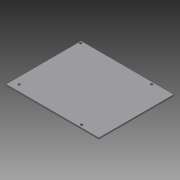
# Autodesk Inventor part: Smoothieboard
Saved by Autodesk Inventor 2014 (Build 180170000, 170)
## iProperties
Created: 2015-02-09
Part Number: Smoothieboard
Material: Generic
Document SubType Name: Modeling
Designer: ThatOtherGuy
Density: 1 g/cm^3
Appearance: Default
Author: ThatOtherGuy
Autodesk Inventor part; units mm, degrees
ref_plane "YZ Plane" through (0, 0, 0) normal (1, 0, 0) x (0, 1, 0)
ref_plane "XZ Plane" through (0, 0, 0) normal (0, 1, 0) x (-1, 0, 0)
ref_plane "XY Plane" through (0, 0, 0) normal (0, 0, 1) x (1, 0, 0)
sketch "Sketch1" plane through (0, 0, 0) normal (0, 0, 1) x (1, 0, 0)
  line L0 (0, 0) -> (129.54, 0)
  line L1 (129.54, 0) -> (129.54, 104.775)
  line L2 (129.54, 104.775) -> (0, 104.775)
  line L3 (0, 104.775) -> (0, 0)
  dimension "d0" = 129.54
  dimension "d1" = 104.775
  constraints: 8 end point, 2 parallel, 1 horizontal, 1 perpendicular
  measures "d0" distance of L0.start L0.end
  measures "d1" distance of L2.end L0.start
extrude "Extrusion1" add sketch "Sketch1" along normal blind 1.6
sketch "Sketch2" plane through (0, 0, 1.6) normal (0, 0, 1) x (1, 0, 0)
  line L0 (0, 0) -> (129.54, 0) projected
  line L1 (0, 104.775) -> (0, 0) projected
  point P0 (9.525, 8.89)
  point P1 (101.6, 3.81)
  point P2 (2.54, 101.6)
  point P3 (101.6, 101.6)
  dimension "d5" = 8.89
  dimension "d6" = 9.525
  dimension "d7" = 3.81
  dimension "d8" = 101.6
  dimension "d9" = 2.54
  dimension "d10" = 101.6
  constraints: 1 horizontal alignment, 1 vertical alignment
  measures "d5" distance from line of point (9.525, 8.89) L0
  measures "d6" distance from line of L1 point (9.525, 8.89)
  measures "d7" distance from line of L0 point (101.6, 3.81)
  measures "d8" distance from line of point (101.6, 3.81) L1
  measures "d9" distance from line of L1 point (2.54, 101.6)
  measures "d10" distance from line of L0 point (2.54, 101.6)
hole "Hole1" at (9.525, 8.89, 1.6) at (101.6, 3.81, 1.6) at (2.54, 101.6, 1.6) at (101.6, 101.6, 1.6) direction (0, 0, -1) diameter 3 end through all
body "Solid1"
